Autodesk Fusion 360 part; units mm, degrees
note: some values were not read from the file. Set by a fixed rule: which sketch regions a step uses.
(part 2 of 2)
sketch "Sketch8" plane through (0, -41.62, 0) normal (0, 1, 0) x (-1, 0, 0)
  line L0 (-53.96, 20) -> (-193.11, 20)
  line L1 (-193.11, 20) -> (-193.11, 0)
  line L2 (-193.11, 0) -> (-53.96, 0)
  line L3 (-53.96, 0) -> (-53.96, 20)
  line L4 (-56.46, 20) -> (-190.61, 20)
  line L5 (-190.61, 20) -> (-190.61, 7)
  line L6 (-190.61, 7) -> (-175.61, 7)
  line L7 (-175.61, 7) -> (-175.61, 2)
  line L8 (-175.61, 2) -> (-71.46, 2)
  line L9 (-71.46, 2) -> (-71.46, 7)
  line L10 (-71.46, 7) -> (-56.46, 7)
  line L11 (-56.46, 7) -> (-56.46, 20)
  line L12 (-183.61, 8.5) -> (-183.61, 12.2929)
  line L13 (-183.61, 12.2929) -> (-179.8171, 8.5)
  line L14 (-179.8171, 8.5) -> (-183.61, 8.5)
  line L15 (-184.61, 18.5) -> (-184.61, 14.7071)
  line L16 (-184.61, 14.7071) -> (-188.4029, 18.5)
  line L17 (-188.4029, 18.5) -> (-184.61, 18.5)
  line L18 (-157.7796, 13) -> (-161.5725, 9.2071)
  line L19 (-161.5725, 9.2071) -> (-161.5725, 13)
  line L20 (-161.5725, 13) -> (-157.7796, 13)
  line L21 (-155.3654, 14) -> (-151.5725, 17.7929)
  line L22 (-151.5725, 17.7929) -> (-151.5725, 14)
  line L23 (-151.5725, 14) -> (-155.3654, 14)
  line L24 (-130.2421, 13) -> (-134.035, 9.2071)
  line L25 (-134.035, 9.2071) -> (-134.035, 13)
  line L26 (-134.035, 13) -> (-130.2421, 13)
  line L27 (-124.035, 17.7929) -> (-124.035, 14)
  line L28 (-124.035, 14) -> (-127.8279, 14)
  line L29 (-127.8279, 14) -> (-124.035, 17.7929)
  line L30 (-119.2421, 13) -> (-123.035, 9.2071)
  line L31 (-123.035, 9.2071) -> (-123.035, 13)
  line L32 (-123.035, 13) -> (-119.2421, 13)
  line L33 (-113.035, 17.7929) -> (-113.035, 14)
  line L34 (-113.035, 14) -> (-116.8279, 14)
  line L35 (-116.8279, 14) -> (-113.035, 17.7929)
  line L36 (-108.2421, 13) -> (-112.035, 9.2071)
  line L37 (-112.035, 9.2071) -> (-112.035, 13)
  line L38 (-112.035, 13) -> (-108.2421, 13)
  line L39 (-105.8279, 14) -> (-102.035, 17.7929)
  line L40 (-102.035, 17.7929) -> (-102.035, 14)
  line L41 (-102.035, 14) -> (-105.8279, 14)
  line L42 (-95.4975, 9.2071) -> (-95.4975, 13)
  line L43 (-95.4975, 13) -> (-91.7046, 13)
  line L44 (-91.7046, 13) -> (-95.4975, 9.2071)
  line L45 (-85.4975, 17.7929) -> (-85.4975, 14)
  line L46 (-85.4975, 14) -> (-89.2904, 14)
  line L47 (-89.2904, 14) -> (-85.4975, 17.7929)
  line L48 (-78.96, 13) -> (-75.1671, 13)
  line L49 (-75.1671, 13) -> (-78.96, 9.2071)
  line L50 (-78.96, 9.2071) -> (-78.96, 13)
  line L51 (-72.7529, 14) -> (-68.96, 17.7929)
  line L52 (-68.96, 17.7929) -> (-68.96, 14)
  line L53 (-68.96, 14) -> (-72.7529, 14)
  line L54 (-63.46, 12.2929) -> (-63.46, 8.5)
  line L55 (-63.46, 8.5) -> (-67.2529, 8.5)
  line L56 (-67.2529, 8.5) -> (-63.46, 12.2929)
  line L57 (-62.46, 14.7071) -> (-62.46, 18.5)
  line L58 (-62.46, 18.5) -> (-58.6671, 18.5)
  line L59 (-58.6671, 18.5) -> (-62.46, 14.7071)
  line L60 (-63.46, 18.5) -> (-63.46, 14.7071)
  line L61 (-63.46, 14.7071) -> (-67.2529, 18.5)
  line L62 (-67.2529, 18.5) -> (-63.46, 18.5)
  line L63 (-62.46, 8.5) -> (-62.46, 12.2929)
  line L64 (-62.46, 12.2929) -> (-58.6671, 8.5)
  line L65 (-58.6671, 8.5) -> (-62.46, 8.5)
  line L66 (-69.6671, 18.5) -> (-73.46, 14.7071)
  line L67 (-73.46, 14.7071) -> (-73.46, 18.5)
  line L68 (-73.46, 18.5) -> (-69.6671, 18.5)
  line L69 (-74.46, 12.2929) -> (-74.46, 8.5)
  line L70 (-74.46, 8.5) -> (-78.2529, 8.5)
  line L71 (-78.2529, 8.5) -> (-74.46, 12.2929)
  line L72 (-89.9975, 14.7071) -> (-89.9975, 18.5)
  line L73 (-89.9975, 18.5) -> (-86.2046, 18.5)
  line L74 (-86.2046, 18.5) -> (-89.9975, 14.7071)
  line L75 (-94.7904, 8.5) -> (-90.9975, 12.2929)
  line L76 (-90.9975, 12.2929) -> (-90.9975, 8.5)
  line L77 (-90.9975, 8.5) -> (-94.7904, 8.5)
  line L78 (-106.535, 14.7071) -> (-106.535, 18.5)
  line L79 (-106.535, 18.5) -> (-102.7421, 18.5)
  line L80 (-102.7421, 18.5) -> (-106.535, 14.7071)
  line L81 (-107.535, 12.2929) -> (-107.535, 8.5)
  line L82 (-107.535, 8.5) -> (-111.3279, 8.5)
  line L83 (-111.3279, 8.5) -> (-107.535, 12.2929)
  line L84 (-113.7421, 18.5) -> (-117.535, 14.7071)
  line L85 (-117.535, 14.7071) -> (-117.535, 18.5)
  line L86 (-117.535, 18.5) -> (-113.7421, 18.5)
  line L87 (-122.3279, 8.5) -> (-118.535, 12.2929)
  line L88 (-118.535, 12.2929) -> (-118.535, 8.5)
  line L89 (-118.535, 8.5) -> (-122.3279, 8.5)
  line L90 (-128.535, 14.7071) -> (-128.535, 18.5)
  line L91 (-128.535, 18.5) -> (-124.7421, 18.5)
  line L92 (-124.7421, 18.5) -> (-128.535, 14.7071)
  line L93 (-129.535, 12.2929) -> (-129.535, 8.5)
  line L94 (-129.535, 8.5) -> (-133.3279, 8.5)
  line L95 (-133.3279, 8.5) -> (-129.535, 12.2929)
  line L96 (-156.0725, 14.7071) -> (-156.0725, 18.5)
  line L97 (-156.0725, 18.5) -> (-152.2796, 18.5)
  line L98 (-152.2796, 18.5) -> (-156.0725, 14.7071)
  line L99 (-157.0725, 12.2929) -> (-157.0725, 8.5)
  line L100 (-157.0725, 8.5) -> (-160.8654, 8.5)
  line L101 (-160.8654, 8.5) -> (-157.0725, 12.2929)
  line L102 (-189.11, 17.7929) -> (-185.3171, 14)
  line L103 (-185.3171, 14) -> (-189.11, 14)
  line L104 (-189.11, 14) -> (-189.11, 17.7929)
  line L105 (-184.61, 12.2929) -> (-184.61, 8.5)
  line L106 (-184.61, 8.5) -> (-188.4029, 8.5)
  line L107 (-188.4029, 8.5) -> (-184.61, 12.2929)
  line L108 (-183.61, 14.7071) -> (-183.61, 18.5)
  line L109 (-183.61, 18.5) -> (-179.8171, 18.5)
  line L110 (-179.8171, 18.5) -> (-183.61, 14.7071)
  line L111 (-157.7796, 14) -> (-161.5725, 14)
  line L112 (-161.5725, 14) -> (-161.5725, 17.7929)
  line L113 (-161.5725, 17.7929) -> (-157.7796, 14)
  line L114 (-151.5725, 13) -> (-151.5725, 9.2071)
  line L115 (-151.5725, 9.2071) -> (-155.3654, 13)
  line L116 (-155.3654, 13) -> (-151.5725, 13)
  line L117 (-130.2421, 14) -> (-134.035, 14)
  line L118 (-134.035, 14) -> (-134.035, 17.7929)
  line L119 (-134.035, 17.7929) -> (-130.2421, 14)
  line L120 (-124.035, 13) -> (-124.035, 9.2071)
  line L121 (-124.035, 9.2071) -> (-127.8279, 13)
  line L122 (-127.8279, 13) -> (-124.035, 13)
  line L123 (-123.035, 17.7929) -> (-119.2421, 14)
  line L124 (-119.2421, 14) -> (-123.035, 14)
  line L125 (-123.035, 14) -> (-123.035, 17.7929)
  line L126 (-116.8279, 13) -> (-113.035, 13)
  line L127 (-113.035, 13) -> (-113.035, 9.2071)
  line L128 (-113.035, 9.2071) -> (-116.8279, 13)
  line L129 (-112.035, 14) -> (-112.035, 17.7929)
  line L130 (-112.035, 17.7929) -> (-108.2421, 14)
  line L131 (-108.2421, 14) -> (-112.035, 14)
  line L132 (-102.035, 9.2071) -> (-105.8279, 13)
  line L133 (-105.8279, 13) -> (-102.035, 13)
  line L134 (-102.035, 13) -> (-102.035, 9.2071)
  line L135 (-95.4975, 14) -> (-95.4975, 17.7929)
  line L136 (-95.4975, 17.7929) -> (-91.7046, 14)
  line L137 (-91.7046, 14) -> (-95.4975, 14)
  line L138 (-85.4975, 13) -> (-85.4975, 9.2071)
  line L139 (-85.4975, 9.2071) -> (-89.2904, 13)
  line L140 (-89.2904, 13) -> (-85.4975, 13)
  line L141 (-78.96, 14) -> (-78.96, 17.7929)
  line L142 (-78.96, 17.7929) -> (-75.1671, 14)
  line L143 (-75.1671, 14) -> (-78.96, 14)
  line L144 (-68.96, 13) -> (-68.96, 9.2071)
  line L145 (-68.96, 9.2071) -> (-72.7529, 13)
  line L146 (-72.7529, 13) -> (-68.96, 13)
  line L147 (-67.96, 13) -> (-64.1671, 13)
  line L148 (-64.1671, 13) -> (-67.96, 9.2071)
  line L149 (-67.96, 9.2071) -> (-67.96, 13)
  line L150 (-57.96, 14) -> (-61.7529, 14)
  line L151 (-61.7529, 14) -> (-57.96, 17.7929)
  line L152 (-57.96, 17.7929) -> (-57.96, 14)
  line L153 (-67.96, 14) -> (-67.96, 17.7929)
  line L154 (-67.96, 17.7929) -> (-64.1671, 14)
  line L155 (-64.1671, 14) -> (-67.96, 14)
  line L156 (-57.96, 13) -> (-57.96, 9.2071)
  line L157 (-57.96, 9.2071) -> (-61.7529, 13)
  line L158 (-61.7529, 13) -> (-57.96, 13)
  line L159 (-74.46, 18.5) -> (-74.46, 14.7071)
  line L160 (-74.46, 14.7071) -> (-78.2529, 18.5)
  line L161 (-78.2529, 18.5) -> (-74.46, 18.5)
  line L162 (-73.46, 8.5) -> (-73.46, 12.2929)
  line L163 (-73.46, 12.2929) -> (-69.6671, 8.5)
  line L164 (-69.6671, 8.5) -> (-73.46, 8.5)
  line L165 (-94.7904, 18.5) -> (-90.9975, 18.5)
  line L166 (-90.9975, 18.5) -> (-90.9975, 14.7071)
  line L167 (-90.9975, 14.7071) -> (-94.7904, 18.5)
  line L168 (-86.2046, 8.5) -> (-89.9975, 8.5)
  line L169 (-89.9975, 8.5) -> (-89.9975, 12.2929)
  line L170 (-89.9975, 12.2929) -> (-86.2046, 8.5)
  line L171 (-107.535, 18.5) -> (-107.535, 14.7071)
  line L172 (-107.535, 14.7071) -> (-111.3279, 18.5)
  line L173 (-111.3279, 18.5) -> (-107.535, 18.5)
  line L174 (-106.535, 12.2929) -> (-102.7421, 8.5)
  line L175 (-102.7421, 8.5) -> (-106.535, 8.5)
  line L176 (-106.535, 8.5) -> (-106.535, 12.2929)
  line L177 (-118.535, 18.5) -> (-118.535, 14.7071)
  line L178 (-118.535, 14.7071) -> (-122.3279, 18.5)
  line L179 (-122.3279, 18.5) -> (-118.535, 18.5)
  line L180 (-117.535, 12.2929) -> (-113.7421, 8.5)
  line L181 (-113.7421, 8.5) -> (-117.535, 8.5)
  line L182 (-117.535, 8.5) -> (-117.535, 12.2929)
  line L183 (-129.535, 14.7071) -> (-133.3279, 18.5)
  line L184 (-133.3279, 18.5) -> (-129.535, 18.5)
  line L185 (-129.535, 18.5) -> (-129.535, 14.7071)
  line L186 (-128.535, 8.5) -> (-128.535, 12.2929)
  line L187 (-128.535, 12.2929) -> (-124.7421, 8.5)
  line L188 (-124.7421, 8.5) -> (-128.535, 8.5)
  line L189 (-157.0725, 14.7071) -> (-160.8654, 18.5)
  line L190 (-160.8654, 18.5) -> (-157.0725, 18.5)
  line L191 (-157.0725, 18.5) -> (-157.0725, 14.7071)
  line L192 (-156.0725, 8.5) -> (-156.0725, 12.2929)
  line L193 (-156.0725, 12.2929) -> (-152.2796, 8.5)
  line L194 (-152.2796, 8.5) -> (-156.0725, 8.5)
  line L195 (-185.3171, 13) -> (-189.11, 9.2071)
  line L196 (-189.11, 9.2071) -> (-189.11, 13)
  line L197 (-189.11, 13) -> (-185.3171, 13)
  line L198 (-179.11, 17.7929) -> (-182.9029, 14)
  line L199 (-179.11, 14) -> (-179.11, 17.7929)
  line L200 (-182.9029, 14) -> (-179.11, 14)
  line L201 (-182.9029, 13) -> (-179.11, 13)
  line L202 (-179.11, 9.2071) -> (-182.9029, 13)
  line L203 (-179.11, 13) -> (-179.11, 9.2071)
  line L204 (-174.3171, 13) -> (-178.11, 13)
  line L205 (-178.11, 13) -> (-178.11, 9.2071)
  line L206 (-178.11, 14) -> (-178.11, 17.7929)
  line L207 (-174.3171, 14) -> (-178.11, 14)
  line L208 (-178.11, 17.7929) -> (-174.3171, 14)
  line L209 (-177.4029, 18.5) -> (-173.61, 14.7071)
  line L210 (-177.4029, 18.5) -> (-173.61, 18.5)
  line L211 (-173.61, 18.5) -> (-173.61, 14.7071)
  line L212 (-178.11, 9.2071) -> (-174.3171, 13)
  line L213 (-177.4029, 8.5) -> (-173.61, 12.2929)
  line L214 (-177.4029, 8.5) -> (-173.61, 8.5)
  line L215 (-173.61, 8.5) -> (-173.61, 12.2929)
  line L216 (-172.61, 8.5) -> (-172.61, 12.2929)
  line L217 (-168.8171, 8.5) -> (-172.61, 8.5)
  line L218 (-168.8171, 8.5) -> (-172.61, 12.2929)
  line L219 (-168.11, 9.2071) -> (-171.9029, 13)
  line L220 (-171.9029, 13) -> (-168.11, 13)
  line L221 (-168.11, 13) -> (-168.11, 9.2071)
  line L222 (-171.9029, 14) -> (-168.11, 14)
  line L223 (-168.11, 14) -> (-168.11, 17.7929)
  line L224 (-168.11, 17.7929) -> (-171.9029, 14)
  line L225 (-168.8171, 18.5) -> (-172.61, 14.7071)
  line L226 (-168.8171, 18.5) -> (-172.61, 18.5)
  line L227 (-172.61, 18.5) -> (-172.61, 14.7071)
  line L228 (-145.035, 17.7929) -> (-141.2421, 14)
  line L229 (-145.035, 14) -> (-145.035, 17.7929)
  line L230 (-141.2421, 14) -> (-145.035, 14)
  line L231 (-144.3279, 18.5) -> (-140.535, 14.7071)
  line L232 (-144.3279, 18.5) -> (-140.535, 18.5)
  line L233 (-140.535, 18.5) -> (-140.535, 14.7071)
  line L234 (-139.535, 18.5) -> (-139.535, 14.7071)
  line L235 (-135.7421, 18.5) -> (-139.535, 18.5)
  line L236 (-135.7421, 18.5) -> (-139.535, 14.7071)
  line L237 (-135.035, 17.7929) -> (-138.8279, 14)
  line L238 (-135.035, 14) -> (-135.035, 17.7929)
  line L239 (-138.8279, 14) -> (-135.035, 14)
  line L240 (-138.8279, 13) -> (-135.035, 13)
  line L241 (-135.035, 9.2071) -> (-138.8279, 13)
  line L242 (-135.035, 13) -> (-135.035, 9.2071)
  line L243 (-135.7421, 8.5) -> (-139.535, 12.2929)
  line L244 (-135.7421, 8.5) -> (-139.535, 8.5)
  line L245 (-139.535, 8.5) -> (-139.535, 12.2929)
  line L246 (-140.535, 8.5) -> (-140.535, 12.2929)
  line L247 (-144.3279, 8.5) -> (-140.535, 8.5)
  line L248 (-144.3279, 8.5) -> (-140.535, 12.2929)
  line L249 (-145.035, 9.2071) -> (-141.2421, 13)
  line L250 (-141.2421, 13) -> (-145.035, 13)
  line L251 (-145.035, 13) -> (-145.035, 9.2071)
extrude "Extrude14" cut sketch "Sketch8" against normal blind 3 contours L12 L13 L14 | L15 L16 L17 | L18 L19 L20 | L21 L22 L23 | L24 L25 L26 | L27 L28 L29 | L30 L31 L32 | L33 L34 L35 | L36 L37 L38 | L39 L40 L41 | L42 L43 L44 | L45 L46 L47 | L48 L49 L50 | L51 L52 L53 | L54 L55 L56 | L57 L58 L59 | L60 L61 L62 | L63 L64 L65 | L66 L67 L68 | L69 L70 L71 | L72 L73 L74 | L75 L76 L77 | L78 L79 L80 | L81 L82 L83 | L84 L85 L86 | L87 L88 L89 | L90 L91 L92 | L93 L94 L95 | L96 L97 L98 | L99 L100 L101 | L102 L103 L104 | L105 L106 L107 | L108 L109 L110 | L111 L112 L113 | L114 L115 L116 | L117 L118 L119 | L120 L121 L122 | L123 L124 L125 | L126 L127 L128 | L129 L130 L131 | L132 L133 L134 | L135 L136 L137 | L138 L139 L140 | L141 L142 L143 | L144 L145 L146 | L147 L148 L149 | L150 L151 L152 | L153 L154 L155 | L156 L157 L158 | L159 L160 L161 | L162 L163 L164 | L165 L166 L167 | L168 L169 L170 | L171 L172 L173 | L174 L175 L176 | L177 L178 L179 | L180 L181 L182 | L183 L184 L185 | L186 L187 L188 | L189 L190 L191 | L192 L193 L194 | L195 L196 L197 | L198 L199 L200 | L201 L202 L203 | L204 L205 L212 | L206 L207 L208 | L209 L210 L211 | L213 L214 L215 | L216 L217 L218 | L219 L220 L221 | L222 L223 L224 | L225 L226 L227
extrude "Extrude15" cut sketch "Sketch8" against normal blind 3 contours L228 L229 L230 | L231 L232 L233 | L234 L235 L236 | L237 L238 L239 | L240 L241 L242 | L243 L244 L245 | L246 L247 L248 | L249 L250 L251
sketch "Sketch9" plane through (0, 0, 0) normal (0, 0, -1) x (1, 0, 0)
  line L0 (53.96, 123.48) -> (53.96, 41.62)
  line L1 (53.96, 41.62) -> (193.11, 41.62)
  line L2 (193.11, 41.62) -> (193.11, 123.48)
  line L3 (193.11, 123.48) -> (53.96, 123.48)
  line L4 (156.1541, 79.706) -> (156.1541, 79.1394)
  line L5 (156.6541, 79.1394) -> (156.1541, 79.1394)
  line L6 (157.117, 79.1394) -> (156.6541, 79.1394)
  line L7 (157.1439, 79.1394) -> (157.117, 79.1394)
  line L8 (157.3409, 79.1394) -> (157.1439, 79.1394)
  line L9 (157.9041, 79.1394) -> (157.3409, 79.1394)
  line L10 (157.9041, 78.3727) -> (157.9041, 79.1394)
  line L11 (157.9041, 78.3727) -> (157.3409, 78.3727)
  line L12 (157.3409, 78.3727) -> (157.1439, 78.3727)
  line L13 (157.1439, 78.3727) -> (157.117, 78.3727)
  line L14 (157.117, 78.3727) -> (156.6541, 78.3727)
  line L15 (156.6541, 78.3727) -> (156.1541, 78.3727)
  line L16 (156.1541, 78.3727) -> (156.1541, 76.8393)
  line L17 (156.6541, 76.8393) -> (156.1541, 76.8393)
  line L18 (157.117, 76.8393) -> (156.6541, 76.8393)
  line L19 (157.1439, 76.8393) -> (157.117, 76.8393)
  line L20 (157.3409, 76.8393) -> (157.1439, 76.8393)
  line L21 (157.9041, 76.8393) -> (157.3409, 76.8393)
  line L22 (157.9041, 76.0726) -> (157.9041, 76.8393)
  line L23 (157.9041, 76.0726) -> (157.3409, 76.0726)
  line L24 (157.3409, 76.0726) -> (157.1439, 76.0726)
  line L25 (157.1439, 76.0726) -> (157.117, 76.0726)
  line L26 (157.117, 76.0726) -> (156.6541, 76.0726)
  line L27 (156.6541, 76.0726) -> (156.1541, 76.0726)
  line L28 (156.1541, 76.0726) -> (156.1541, 74.5392)
  line L29 (156.6541, 74.5392) -> (156.1541, 74.5392)
  line L30 (157.117, 74.5392) -> (156.6541, 74.5392)
  line L31 (157.1439, 74.5392) -> (157.117, 74.5392)
  line L32 (157.3409, 74.5392) -> (157.1439, 74.5392)
  line L33 (157.9041, 74.5392) -> (157.3409, 74.5392)
  line L34 (157.9041, 73.7725) -> (157.9041, 74.5392)
  line L35 (157.9041, 73.7725) -> (157.3409, 73.7725)
  line L36 (157.3409, 73.7725) -> (157.1439, 73.7725)
  line L37 (157.1439, 73.7725) -> (157.117, 73.7725)
  line L38 (157.117, 73.7725) -> (156.6541, 73.7725)
  line L39 (156.6541, 73.7725) -> (156.1541, 73.7725)
  line L40 (156.1541, 73.7725) -> (156.1541, 73.206)
  line L41 (156.1541, 73.206) -> (152.6541, 73.206)
  line L42 (152.6541, 73.206) -> (152.6541, 75.3059)
  line L43 (152.1541, 75.3059) -> (152.6541, 75.3059)
  line L44 (151.6912, 75.3059) -> (152.1541, 75.3059)
  line L45 (151.6643, 75.3059) -> (151.6912, 75.3059)
  line L46 (151.4673, 75.3059) -> (151.6643, 75.3059)
  line L47 (150.9041, 75.3059) -> (151.4673, 75.3059)
  line L48 (150.9041, 77.606) -> (150.9041, 75.3059)
  line L49 (150.9041, 77.606) -> (151.4673, 77.606)
  line L50 (151.4673, 77.606) -> (151.6643, 77.606)
  line L51 (151.6643, 77.606) -> (151.6912, 77.606)
  line L52 (151.6912, 77.606) -> (152.1541, 77.606)
  line L53 (152.1541, 77.606) -> (152.6541, 77.606)
  line L54 (152.6541, 77.606) -> (152.6541, 79.706)
  line L55 (152.6541, 79.706) -> (156.1541, 79.706)
  line L56 (150, 81.1423) -> (160, 81.1423)
  line L57 (160, 81.1423) -> (160, 71.1423)
  line L58 (160, 71.1423) -> (150, 71.1423)
  line L59 (150, 71.1423) -> (150, 81.1423)
  line L60 (140, 61.1423) -> (140, 91.1423)
  line L61 (140, 91.1423) -> (170, 91.1423)
  line L62 (170, 91.1423) -> (170, 61.1423)
  line L63 (170, 61.1423) -> (140, 61.1423)
  line L64 (150, 81.1423) -> (150, 91.1423)
  line L65 (160, 81.1423) -> (160, 91.1423)
  line L66 (160, 81.1423) -> (170, 81.1423)
  line L67 (160, 71.1423) -> (170, 71.1423)
  line L68 (160, 71.1423) -> (160, 61.1423)
  line L69 (150, 71.1423) -> (150, 61.1423)
  line L70 (150, 61.1423) -> (150, 71.1423)
  line L71 (150, 71.1423) -> (140, 71.1423)
  line L72 (150, 81.1423) -> (140, 81.1423)
  line L73 (169, 62.1423) -> (141, 62.1423)
  line L74 (141, 62.1423) -> (141, 90.1423)
  line L75 (141, 90.1423) -> (169, 90.1423)
  line L76 (169, 90.1423) -> (169, 62.1423)
  line L77 (149, 82.1423) -> (140, 82.1423)
  line L78 (149, 82.1423) -> (149, 91.1423)
  line L79 (159, 82.1423) -> (159, 91.1423)
  line L80 (151, 82.1423) -> (159, 82.1423)
  line L81 (151, 82.1423) -> (151, 91.1423)
  line L82 (161, 82.1423) -> (170, 82.1423)
  line L83 (161, 82.1423) -> (161, 91.1423)
  line L84 (161, 72.1423) -> (170, 72.1423)
  line L85 (161, 80.1423) -> (161, 72.1423)
  line L86 (161, 80.1423) -> (170, 80.1423)
  line L87 (161, 70.1423) -> (170, 70.1423)
  line L88 (161, 70.1423) -> (161, 61.1423)
  line L89 (159, 70.1423) -> (150, 70.1423)
  line L90 (159, 70.1423) -> (159, 61.1423)
  line L91 (151, 71.1423) -> (151, 61.1423)
  arc A0 (149, 61.1423) -> (151, 61.1423) centre (150, 61.1423) ccw
  line L92 (149, 61.1423) -> (149, 71.1423)
  arc A1 (151, 71.1423) -> (149, 71.1423) centre (150, 71.1423) ccw
  line L93 (150, 70.1423) -> (140, 70.1423)
  line L94 (150, 80.1423) -> (140, 80.1423)
  line L95 (149, 71.1423) -> (149, 81.1423)
  line L96 (150, 72.1423) -> (140, 72.1423)
  line L97 (150, 80.1423) -> (160, 80.1423)
  line L98 (159, 82.1423) -> (159, 71.1423)
  line L99 (150, 72.1423) -> (161, 72.1423)
  line L100 (151, 82.1423) -> (151, 71.1423)
  dimension "d103" = 10
  dimension "d104" = -10
  dimension "d105" = 1
  dimension "d106" = -1
  dimension "d107" = -1
  dimension "d108" = 1
  dimension "d109" = 1
  dimension "d110" = -1
  dimension "d111" = 1
  dimension "d112" = -1
  dimension "d113" = -1
  dimension "d114" = -1
  dimension "d115" = -1
  dimension "d116" = 1
  constraint horizontal L56
  constraint vertical L57
  constraint horizontal L58
  constraint vertical L59
  constraint coincident L61 L64.end
  constraint perpendicular L61 L64
  constraint coincident L61 L65.end
  constraint perpendicular L61 L65
  constraint coincident L62 L66.end
  constraint perpendicular L62 L66
  constraint coincident L62 L67.end
  constraint perpendicular L62 L67
  constraint coincident L63 L68.end
  constraint perpendicular L63 L68
  constraint coincident L63 L69.end
  constraint perpendicular L63 L69
  constraint coincident L60 L71.end
  constraint perpendicular L60 L71
  constraint coincident L60 L72.end
  constraint perpendicular L60 L72
  constraint coincident L57 L97.end
  constraint perpendicular L57 L97
  constraint coincident L58 L98.end
  constraint perpendicular L58 L98
  constraint tangent A1 L100
  measures "d103" distance of L56.start L58.end
  measures "d104" distance of L57
extrude "Extrude16" cut sketch "Sketch9" against normal blind 2 contours L4 L5 L6 L7 L8 L9 L10 L11 L12 L13 L14 L15 L16 L17 L18 L19 L20 L21 L22 L23 L24 L25 L26 L27 L28 L29 L30 L31 L32 L33 L34 L35 L36 L37 L38 L39 L40 L41 L42 L43 L44 L45 L46 L47 L49 L50 L51 L52 L53 L54 L55 L97 L98 L99 L100 | L4 L5 L6 L7 L8 L9 L10 L11 L12 L13 L14 L15 L16 L17 L18 L19 L20 L21 L22 L23 L24 L25 L26 L27 L28 L29 L30 L31 L32 L33 L34 L35 L36 L37 L38 L39 L40 L41 L42 L43 L44 L45 L46 L47 L49 L50 L51 L52 L53 L54 L55 L100 | L74 L94 L95 L96 | L75 L79 L80 L81 | L73 L89 L90 L91 | L73 L74 L92 L93 | L74 L75 L77 L78 | L76 L84 L85 L86 | L75 L76 L82 L83 | L73 L76 L87 L88
